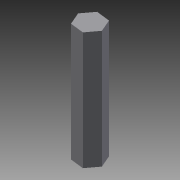
# Autodesk Inventor part: rod2
Saved by Autodesk Inventor 2016 (Build 200138000, 138)
## iProperties
Created: 2016-01-27
Part Number: rod2
Material: Generic
Document SubType Name: Modeling
Designer: 278648
Density: 1 g/cm^3
Appearance: Default
Author: 278648
Autodesk Inventor part; units mm, degrees
ref_plane "YZ Plane" through (0, 0, 0) normal (1, 0, 0) x (0, 1, 0)
ref_plane "XZ Plane" through (0, 0, 0) normal (0, 1, 0) x (-1, 0, 0)
ref_plane "XY Plane" through (0, 0, 0) normal (0, 0, 1) x (1, 0, 0)
sketch "Sketch1" plane through (0, 0, 0) normal (0, 1, 0) x (-1, 0, 0)
  line L0 (-4.3994, -5.8659) -> (-7.2797, 0.8771)
  line L1 (-7.2797, 0.8771) -> (-2.8803, 6.7429)
  line L2 (-2.8803, 6.7429) -> (4.3994, 5.8659)
  line L3 (4.3994, 5.8659) -> (7.2797, -0.8771)
  line L4 (7.2797, -0.8771) -> (2.8803, -6.7429)
  line L5 (2.8803, -6.7429) -> (-4.3994, -5.8659)
  point P0 (0, 0)
  point P1 (0, 0)
  dimension "d0" = 12.7
  constraints: 12 end point, 1 coincident, 13 other
  measures "d0" distance between parallel lines of L2 L5
extrude "Extrusion1" add sketch "Sketch1" along normal blind 76.2
body "Solid1"
